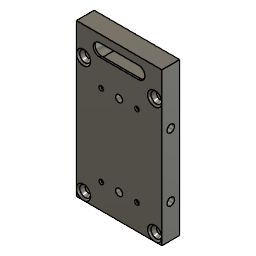
suction pump head (Autodesk Fusion 360 archive; units mm, degrees)
design "tool changer head"
Autodesk Fusion 360 part; units mm, degrees
sketch "Sketch1" plane through (0, 0, 0) normal (0, 0, 1) x (1, 0, 0)
  line L0 (24, 36.75) -> (-24, 36.75)
  line L1 (-24, 36.75) -> (-24, -36.75)
  line L2 (-24, -36.75) -> (24, -36.75)
  line L3 (24, -36.75) -> (24, 36.75)
  line L4 (24, 36.75) -> (-24, -36.75) construction
  line L5 (-24, 36.75) -> (24, -36.75) construction
  line L6 (-24, 36.75) -> (-20, 36.75)
  line L7 (-20, 36.75) -> (-20, 32.75)
  line L8 (-20, 32.75) -> (-24, 32.75)
  line L9 (-24, 32.75) -> (-24, 36.75)
  line L10 (24, 36.75) -> (20, 36.75)
  line L11 (20, 36.75) -> (20, 32.75)
  line L12 (20, 32.75) -> (24, 32.75)
  line L13 (24, 32.75) -> (24, 36.75)
  line L14 (24, -36.75) -> (20, -36.75)
  line L15 (20, -36.75) -> (20, -32.75)
  line L16 (20, -32.75) -> (24, -32.75)
  line L17 (24, -32.75) -> (24, -36.75)
  line L18 (-24, -36.75) -> (-20, -36.75)
  line L19 (-20, -36.75) -> (-20, -32.75)
  line L20 (-20, -32.75) -> (-24, -32.75)
  line L21 (-24, -32.75) -> (-24, -36.75)
  circle A0 centre (-20, 32.75) radius 2
  circle A1 centre (20, 32.75) radius 2
  circle A2 centre (-20, -32.75) radius 2
  circle A3 centre (20, -32.75) radius 2
  line L22 (0, 36.75) -> (0, 22.75)
  circle A4 centre (0, 22.75) radius 1.95
  line L23 (0, -36.75) -> (0, -22.75)
  circle A5 centre (0, -22.75) radius 1.95
  line L24 (0, -36.75) -> (0, 0)
  line L25 (10, 22.75) -> (-10, 22.75)
  line L26 (-10, 22.75) -> (-10, -22.75)
  line L27 (-10, -22.75) -> (10, -22.75)
  line L28 (10, -22.75) -> (10, 22.75)
  line L29 (10, 22.75) -> (-10, -22.75) construction
  line L30 (-10, 22.75) -> (10, -22.75) construction
  circle A6 centre (-10, 22.75) radius 0.5
  circle A7 centre (-10, 22.75) radius 1.25
  circle A8 centre (10, 22.75) radius 0.5
  circle A9 centre (10, 22.75) radius 1.25
  circle A10 centre (-10, -22.75) radius 0.5
  circle A11 centre (-10, -22.75) radius 1.25
  circle A12 centre (10, -22.75) radius 0.5
  circle A13 centre (10, -22.75) radius 1.25
  dimension "d1" = 48
  dimension "d2" = 73.5
  dimension "d3" = 4
  dimension "d4" = 4
  dimension "d5" = 4
  dimension "d6" = 4
  dimension "d7" = 4
  dimension "d8" = 4
  dimension "d9" = 4
  dimension "d10" = 4
  dimension "d11" = 4
  dimension "d12" = 4
  dimension "d13" = 4
  dimension "d14" = 4
  dimension "d15" = 14
  dimension "d16" = 3.9
  dimension "d17" = 14
  dimension "d18" = 3.9
  dimension "d29" = 36.75
  dimension "d30" = 20
  dimension "d31" = 45.5
  dimension "d32" = 1
  dimension "d33" = 2.5
  dimension "d34" = 1
  dimension "d35" = 2.5
  dimension "d36" = 1
  dimension "d37" = 2.5
  dimension "d38" = 1
  dimension "d39" = 2.5
  constraint horizontal L0
  constraint perpendicular L0 L1
  constraint parallel L0 L2
  constraint parallel L1 L3
  constraint coincident L4 L24.end
  constraint coincident L5 L24.end
  constraint coincident L24.end origin
  constraint horizontal L6
  constraint vertical L7
  constraint horizontal L8
  constraint vertical L9
  constraint horizontal L10
  constraint vertical L11
  constraint horizontal L12
  constraint vertical L13
  constraint horizontal L14
  constraint vertical L15
  constraint horizontal L16
  constraint vertical L17
  constraint horizontal L18
  constraint vertical L19
  constraint horizontal L20
  constraint vertical L21
  constraint coincident L7.end L8.start
  constraint coincident L11.end L12.start
  constraint coincident L19.end L20.start
  constraint coincident L15.end L16.start
  constraint midpoint L0 L22.start
  constraint perpendicular L0 L22
  constraint coincident L22.end A4.centre
  constraint midpoint L2 L23.start
  constraint perpendicular L2 L23
  constraint coincident L23.end A5.centre
  constraint perpendicular L2 L24
  constraint horizontal L25
  constraint perpendicular L25 L26
  constraint parallel L25 L27
  constraint parallel L26 L28
  constraint coincident L29 L24.end
  constraint coincident L30 L24.end
  constraint coincident L25.end L26.start
  constraint coincident L25.start L28.end
  constraint concentric A8 A9
  constraint coincident L26.end L27.start
  constraint concentric A10 A11
  constraint coincident L27.end L28.start
  measures "d1" distance of L1.end L2.end
  measures "d2" distance of L0.end L1.end
  measures "d3" distance of L0.end L6.end
  measures "d4" distance of L0.end L8.end
  measures "d5" distance of L0.start L10.end
  measures "d6" distance of L0.start L12.end
  measures "d7" distance of L2.end L14.end
  measures "d8" distance of L2.end L16.end
  measures "d9" distance of L1.end L18.end
  measures "d10" distance of L1.end L20.end
  measures "d11" diameter of A0
  measures "d12" diameter of A1
  measures "d13" diameter of A2
  measures "d14" diameter of A3
  measures "d15" distance of L22.start L22.end
  measures "d16" diameter of A4
  measures "d17" distance of L23.start L23.end
  measures "d18" diameter of A5
  measures "d29" distance of L23.start L24.end
  measures "d30" distance of L26.end L27.end
  measures "d31" distance of L25.end L26.end
  measures "d32" diameter of A6
  measures "d33" diameter of A7
  measures "d34" diameter of A8
  measures "d35" diameter of A9
  measures "d36" diameter of A10
  measures "d37" diameter of A11
  measures "d38" diameter of A12
  measures "d39" diameter of A13
extrude "Extrude1" add sketch "Sketch1" along normal blind 10 contours L0 L3 L10 L11 L12 L13 A1 | L0 L2 L3 L11 L12 L15 L16 A1 A3 L22 A4 L23 A5 L24 L25 L27 L28 A9 A13 | L0 L1 L2 L7 L8 L19 L20 A0 A2 L22 A4 L23 A5 L24 L25 L26 L27 A7 A11 | L2 L3 L14 L15 L16 L17 A3 | L0 L1 L6 L7 L8 L9 A0 | A4 A5 L25 L26 L27 L28 A7 A9 A11 A13 | L25 L28 A8 A9 | L25 L28 A8 A9 | L25 L26 A6 A7 | L25 L26 A6 A7 | L1 L2 L18 L19 L20 L21 A2 | L25 L28 A8 | L25 L28 A8 | L25 L26 A6 | L25 L26 A6 | L27 L28 A12 A13 | L27 L28 A12 A13 | L26 L27 A10 A11 | L26 L27 A10 A11 | L27 L28 A12 | L27 L28 A12 | L26 L27 A10 | L26 L27 A10 makes body 1
sketch "Sketch2" plane through (24, 0, 0) normal (1, 0, 0) x (0, 0, -1)
  line L0 (0, -36.75) -> (0, 36.75)
  line L1 (0, 36.75) -> (-10, 36.75)
  line L2 (-10, 36.75) -> (-10, -36.75)
  line L3 (-10, -36.75) -> (0, -36.75)
  line L4 (-5, 36.75) -> (-5, 17.75)
  line L5 (-5, -36.75) -> (-5, -17.75)
  circle A0 centre (-5, -17.75) radius 2.1
  circle A1 centre (-5, 17.75) radius 2.1
  dimension "d21" = 19
  dimension "d22" = 19
  dimension "d23" = 4.2
  dimension "d24" = 4.2
  constraint midpoint L1 L4.start
  constraint perpendicular L1 L4
  constraint midpoint L3 L5.start
  constraint perpendicular L3 L5
  constraint coincident L5.end A0.centre
  constraint coincident L4.end A1.centre
  measures "d21" distance of L4.start L4.end
  measures "d22" distance of L5.start L5.end
  measures "d23" diameter of A0
  measures "d24" diameter of A1
extrude "Extrude2" cut sketch "Sketch2" against normal blind 48 contours A0 | A1 bodies 1
chamfer "Chamfer1" distance 2 angle 45 6 edges at (24, 18.5094, 6.9579) (24, -16.9906, 6.9579) (18.1353, -32.0268, 10) (18.1353, 33.4732, 10) (-21.8647, 33.4732, 10) (-21.8647, -32.0268, 10) on bodies 1
extrude "Extrude3" cut sketch "Sketch1" along normal blind 10 contours L25 L28 A8 | L25 L28 A8 | L25 L26 A6 | L25 L26 A6 | L27 L28 A12 | L27 L28 A12 | L26 L27 A10 | L26 L27 A10 bodies 1
extrude "Extrude4" cut sketch "Sketch1" along normal blind 10 and the other way blind -9 contours L25 L28 A8 A9 | L25 L28 A8 A9 | L25 L26 A6 A7 | L25 L26 A6 A7 | L27 L28 A12 A13 | L27 L28 A12 A13 | L26 L27 A10 A11 | L26 L27 A10 A11 bodies 1
extrude "Extrude5" add 1 faces at (6.6667, 36.75, 3.3333) along direction (0, 1, 0) blind 12 on bodies 1 bodies 1
sketch "Sketch3" plane through (0, 0, 10) normal (0, 0, 1) x (1, 0, 0)
  circle A0 centre (0, 22.75) radius 1.95
  line L0 (-24, 32.75) -> (-24, -32.75)
  line L1 (24, -32.75) -> (24, 32.75)
  line L2 (24, 48.75) -> (-24, 48.75)
  line L3 (-24, 48.75) -> (24, 48.75)
  line L4 (24, 48.75) -> (24, 36.75)
  line L5 (24, 36.75) -> (-24, 36.75)
  line L6 (-24, 36.75) -> (-24, 48.75)
  line L7 (0, 36.75) -> (0, 41)
  line L8 (11, 36.5) -> (-11, 36.5)
  line L9 (-11, 36.5) -> (-11, 45.5)
  line L10 (-11, 45.5) -> (11, 45.5)
  line L11 (11, 45.5) -> (11, 36.5)
  line L12 (11, 36.5) -> (-11, 45.5) construction
  line L13 (-11, 36.5) -> (11, 45.5) construction
  circle A1 centre (11, 41) radius 4.5
  circle A2 centre (-11, 41) radius 4.5
  line L14 (11, 44.5) -> (-11, 44.5)
  line L15 (-11, 44.5) -> (-11, 37.5)
  line L16 (-11, 37.5) -> (11, 37.5)
  line L17 (11, 37.5) -> (11, 44.5)
  line L18 (11, 44.5) -> (-11, 37.5) construction
  line L19 (-11, 44.5) -> (11, 37.5) construction
  circle A3 centre (11, 41) radius 3.5
  circle A4 centre (-11, 41) radius 3.5
  circle A5 centre (-10, 22.75) radius 1.25
  circle A6 centre (-10, -22.75) radius 1.25
  circle A7 centre (10, 22.75) radius 1.25
  circle A8 centre (10, -22.75) radius 1.25
  circle A9 centre (0, -22.75) radius 1.95
  line L20 (-20, -36.75) -> (20, -36.75)
  arc A10 (-20, -36.75) -> (-24, -32.75) centre (-20, -32.75) ccw
  arc A11 (24, -32.75) -> (20, -36.75) centre (20, -32.75) ccw
  circle A12 centre (-20, 32.75) radius 4
  circle A13 centre (20, 32.75) radius 4
  line L21 (24, 32.75) -> (24, 48.75)
  line L22 (-24, 48.75) -> (-24, 32.75)
  point P0 (0, 41)
  point P1 (0, 41)
  dimension "d49" = 12
  dimension "d50" = 4.25
  dimension "d51" = 22
  dimension "d52" = 9
  dimension "d53" = 7
  constraint horizontal L3
  constraint vertical L4
  constraint horizontal L5
  constraint vertical L6
  constraint coincident L2.end L3.start
  constraint midpoint L5 L7.start
  constraint perpendicular L5 L7
  constraint horizontal L8
  constraint perpendicular L8 L9
  constraint parallel L8 L10
  constraint parallel L9 L11
  constraint coincident L12 P1
  constraint coincident L13 P1
  constraint coincident P1 P0
  constraint midpoint L11 A1.centre
  constraint coincident L10.end A1
  constraint midpoint L9 A2.centre
  constraint coincident L9.end A2
  constraint horizontal L14
  constraint perpendicular L14 L15
  constraint parallel L14 L16
  constraint parallel L15 L17
  constraint coincident L18 P1
  constraint coincident L19 P1
  constraint concentric A1 A3
  constraint coincident L14.start A3
  constraint tangent L14 A3
  constraint concentric A2 A4
  constraint coincident L14.end A4
  measures "d49" distance of L2.end L5.end
  measures "d50" distance of L7.start P1
  measures "d51" distance of L9.end L10.end
  measures "d52" distance of L8.end L9.end
  measures "d53" distance of L14.end L15.end
extrude "Extrude6" cut sketch "Sketch3" against normal blind 10 contours L9 L15 A4 | A2 L14 L16 A4 | L9 L15 A4 | A1 A2 L14 L16 | L11 L17 A3 | A1 L14 L16 A3 | L11 L17 A3 bodies 1
extrude "Extrude7" cut sketch "Sketch3" along normal blind -1 and the other way blind 10 contours L5 L9 A2 A4 | L5 L9 A2 | L5 L9 A2 L16 | L5 L9 A2 | L9 A2 L14 | L10 A1 A2 L14 | L5 L8 A1 A2 | L5 L7 A2 L16 | L5 L11 A1 A3 | L11 A1 L14 | L5 L11 A1 | L5 L11 A1 | L5 L7 A1 L16 | L5 L11 A1 L16 bodies 1
sketch "Sketch4" plane through (24, 0, 0) normal (1, 0, 0) x (0, 0, -1)
  line L0 (0, -36.75) -> (0, 48.75)
  line L1 (0, 48.75) -> (-10, 48.75)
  line L2 (-5, 48.75) -> (-5, 41)
  circle A0 centre (-5, 41) radius 4
  circle A1 centre (-5, 17.75) radius 4.1
  line L3 (-10, 48.75) -> (-10, 32.75)
  line L4 (-10, -36.75) -> (0, -36.75)
  circle A2 centre (-5, -17.75) radius 4.1
  line L5 (-10, 32.75) -> (-10, -32.75)
  line L6 (-10, -32.75) -> (-10, -36.75)
  dimension "d60" = 7.75
  dimension "d61" = 8
  constraint midpoint L1 L2.start
  constraint perpendicular L1 L2
  constraint coincident L2.end A0.centre
  measures "d60" distance of L2.start L2.end
  measures "d61" diameter of A0
extrude "Extrude8" cut sketch "Sketch4" against normal blind 6.5 contours A0 bodies 1
chamfer "Chamfer2" distance 1.5 distance2 1 6 edges at (22, 18.5094, 6.9579) (22, -16.9906, 6.9579) (18.1353, -32.0268, 8) (-21.8647, -32.0268, 8) (-21.8647, 33.4732, 8) (18.1353, 33.4732, 8) measured on face at (23.5556, 19.3361, 1.7065) measured on face at (23.5556, -15.2636, 2.3203) measured on face at (23.5163, -32.2228, 9.5556) measured on face at (-20.2657, -29.2044, 9.5556) measured on face at (-22.2169, 35.5298, 9.5556) measured on face at (17.7831, 35.5298, 9.5556) on bodies 1
mirror "Mirror1" about plane through (24, 36.75, 0) normal (1, 0, 0) of bodies 1 makes body 2
move_body "Move1" bodies 2 to x (1, 0, 0) y (0, 1, 0) z (0, 0, 1) at (-48, 0, 0)
hidden bodies 1
equation "d2 = 17.5 mm + ( ( 2 * 8 ) * 1 mm ) + 4 * ( d15 - ( 8 / 2 ) * 1 mm - 0 mm )"
equation "d4 = d3"
equation "d5 = d4"
equation "d6 = d4"
equation "d7 = d4"
equation "d8 = d4"
equation "d9 = d4"
equation "d10 = d4"
equation "d12 = d11"
equation "d13 = d11"
equation "d14 = d11"
equation "d17 = d15"
equation "d18 = d16"
equation "d21 = 14 mm + 1 mm + 4 mm"
equation "d22 = d21"
equation "d29 = d2 / 2"
equation "d50 = ( 8.5 / 2 ) * 1 mm"
